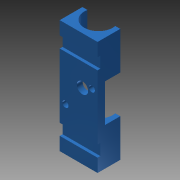
# Autodesk Inventor part: Linear bearing 8mm clamp
Saved by Autodesk Inventor 2013 SP2 (Build 170200200, 200)
## iProperties
Created: 2017-03-11
Part Number: Linear bearing 8mm clamp
Material: Generic
Document SubType Name: Modeling
Designer: Herman de Vries
Density: 1 g/cm^3
Mass: 9.50106 g
Surface Area: 48.9856 cm^2
Volume: 9.50106 cm^3
Author: Herman de Vries
Autodesk Inventor part; units mm, degrees
ref_plane "YZ Plane" through (0, 0, 0) normal (1, 0, 0) x (0, 1, 0)
ref_plane "XZ Plane" through (0, 0, 0) normal (0, 1, 0) x (-1, 0, 0)
ref_plane "XY Plane" through (0, 0, 0) normal (0, 0, 1) x (1, 0, 0)
sketch "Sketch1" plane through (0, 0, 0) normal (0, 0, 1) x (1, 0, 0)
  line L0 (0, 0) -> (20, 0)
  line L1 (20, 0) -> (20, 12)
  line L2 (20, 12) -> (0, 12) construction
  line L3 (0, 12) -> (0, 0)
  arc A0 (2.6515, 12) -> (17.3485, 12) centre (10, 10.5) ccw
  line L4 (0, 12) -> (2.6515, 12)
  line L5 (17.3485, 12) -> (20, 12)
  point P0 (10, 12)
  dimension "d0" = 20
  dimension "d1" = 12
  dimension "d2" = 15
  dimension "d14" = 1.5
  constraints: 12 end point, 2 collinear, 2 parallel, 2 point on circle, 2 point on line, 1 centre point, 1 horizontal, 1 midpoint, 1 perpendicular, 1 vertical alignment
  measures "d0" distance of L2.end L1.end
  measures "d1" distance of L0.end L1.end
  measures "d2" diameter of A0
  measures "d14" distance of A0.centre point (10, 12)
extrude "Extrusion1" add sketch "Sketch1" along normal blind 60
sketch "Sketch4" plane through (0, 12, 0) normal (0, 1, 0) x (1, 0, 0)
  line L0 (0, -20) -> (20, -20)
  line L1 (20, -20) -> (20, -40)
  line L2 (20, -40) -> (0, -40)
  line L3 (0, -40) -> (0, -20)
  line L4 (0, 0) -> (0, -60) projected
  line L5 (17.5, 0) -> (2.5, 0) projected
  line L6 (20, 0) -> (20, -60) projected
  point P0 (0, -30)
  point P1 (0, -30)
  point P2 (10, -20)
  point P3 (10, 0)
  point P4 (17.3485, 0)
  point P5 (2.6515, 0)
  dimension "d15" = 20
  constraints: 8 end point, 4 midpoint, 2 parallel, 1 coincident, 1 collinear, 1 horizontal, 1 perpendicular, 1 vertical alignment
  measures "d15" distance of L2.end L0.start
extrude "Extrusion4" cut sketch "Sketch4" against normal blind 8
sketch "Sketch5" plane through (0, 4, 0) normal (0, 1, 0) x (1, 0, 0)
  circle A0 centre (3, -23) radius 1.6
  circle A1 centre (17, -37) radius 1.6
  line L0 (17, -37) -> (3, -37) construction
  line L1 (3, -37) -> (3, -23) construction
  line L2 (3, -23) -> (17, -23) construction
  line L3 (17, -23) -> (17, -37) construction
  line L4 (0, -40) -> (0, -20) construction
  line L5 (17.5, 0) -> (2.5, 0) construction
  line L6 (6.2583, -40) -> (2.5, -40) construction
  circle A2 centre (12, -35) radius 1.6 construction
  circle A3 centre (12, -35) radius 3
  point P0 (0, 0)
  point P1 (3, -30)
  point P2 (0, -30)
  point P3 (10, -23)
  point P4 (10, 0)
  point P5 (17.3485, 0)
  point P6 (2.6515, 0)
  point P7 (17.3485, -40)
  point P8 (2.6515, -40)
  dimension "d19" = 3.2
  dimension "d20" = 3.2
  dimension "d21" = 3
  dimension "d22" = 3
  dimension "d30" = 6
  constraints: 8 end point, 4 midpoint, 3 centre point, 2 parallel, 1 coincident, 1 horizontal, 1 horizontal alignment, 1 perpendicular, 1 vertical alignment
  measures "d19" diameter of A0
  measures "d20" diameter of A1
  measures "d21" distance between parallel lines of L4 L1
  measures "d22" distance from line of L0.end L6
  measures "d30" diameter of A3
extrude "Extrusion5" cut sketch "Sketch5" against normal blind 10
sketch "Sketch6" plane through (0, 0, 0) normal (-1, 0, 0) x (0, 0, 1)
  line L0 (7, 0) -> (13, 0)
  line L1 (13, 0) -> (13, 1.5)
  line L2 (13, 1.5) -> (7, 1.5)
  line L3 (7, 1.5) -> (7, 0)
  line L4 (47, 0) -> (53, 0)
  line L5 (53, 0) -> (53, 1.5)
  line L6 (53, 1.5) -> (47, 1.5)
  line L7 (47, 1.5) -> (47, 0)
  line L8 (0, 12) -> (20, 12) construction
  line L9 (40, 12) -> (60, 12) construction
  point P0 (0, 0)
  point P1 (10, 1.5)
  point P2 (10, 12)
  point P3 (50, 1.5)
  point P4 (50, 12)
  dimension "d25" = 6
  dimension "d26" = 1.5
  dimension "d27" = 6
  constraints: 16 end point, 4 midpoint, 4 parallel, 2 horizontal, 2 horizontal alignment, 2 perpendicular, 2 vertical alignment, 1 collinear
  measures "d25" distance of L2.end L1.end
  measures "d26" distance of L1.end L0.end
  measures "d27" distance of L6.end L5.end
extrude "Extrusion6" cut sketch "Sketch6" against normal through all
equation "\"d20\" = d19"
body "Solid1"
